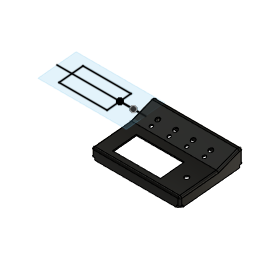
F24-Top (Autodesk Fusion 360 design; units mm, degrees)
Autodesk Fusion 360 part; units mm, degrees
sketch "Sketch1" plane through (0, 0, 0) normal (1, 0, 0) x (0, 1, 0)
  line L0 (49.5653, 19.5568) -> (20.1722, 19.5568)
  line L1 (-50.4347, -6.4432) -> (49.5653, -6.4432)
  line L2 (49.5653, 3.5568) -> (-50.4347, -6.4432)
  line L3 (20.1722, 19.5568) -> (20.1722, 28.5568)
  line L4 (44.5653, 26.5568) -> (43.5653, 26.5568)
  line L5 (-50.4347, 19.5568) -> (-50.4347, -6.4432)
  line L6 (20.1722, 19.5568) -> (10.0727, 15.6075)
  line L7 (49.5653, -6.4432) -> (-15.6066, -6.4432)
  line L8 (67.3511, 38.0053) -> (20.1722, 19.5568)
  line L9 (10.5451, 13.6448) -> (-45.4347, 8.0468)
  line L10 (43.5653, 26.5568) -> (10.5451, 13.6448)
  line L11 (20.1722, 28.5568) -> (49.5653, 28.5568)
  line L12 (44.5653, 3.0568) -> (44.5653, 26.5568)
  line L13 (-15.6066, -6.4432) -> (-15.6066, -63.0186)
  line L14 (49.5653, 19.5568) -> (-50.4347, 9.5568)
  line L15 (-45.4347, 8.0468) -> (-45.4347, -5.9432)
  line L16 (49.5653, 28.5568) -> (49.5653, 19.5568)
  line L17 (49.5653, 19.5568) -> (-50.4347, 19.5568)
  line L18 (49.5653, -6.4432) -> (49.5653, 19.5568)
  line L19 (49.5653, -63.0186) -> (49.5653, -6.4432)
  line L20 (-15.6066, -63.0186) -> (49.5653, -63.0186)
  line L21 (-15.6066, -6.4432) -> (-63.7664, -6.4432)
  line L22 (-63.7664, -6.4432) -> (-63.7664, -63.0262)
  line L23 (-63.7664, -63.0262) -> (-15.6066, -63.0262)
  line L24 (-15.6066, -63.0262) -> (-15.6066, -6.4432)
  line L25 (53.9927, 48.0645) -> (16.8652, 48.0645)
  line L26 (16.8652, 48.0645) -> (16.8652, 28.5568)
  line L27 (16.8652, 28.5568) -> (53.9927, 28.5568)
  line L28 (53.9927, 28.5568) -> (53.9927, 48.0645)
  point P0 (34.5128, -10.5651)
  dimension "d1" = 10
  dimension "d2" = 10
  dimension "d3" = 16
  dimension "d5" = 9
  dimension "d9" = 5
  dimension "d10" = 2
  dimension "d12" = 2
  dimension "d13" = 2
  dimension "d15" = 5
  dimension "d99" = 100
  dimension "d100" = 1
  dimension "d84" = 65.172
  constraint horizontal L17
  constraint vertical L5
  constraint horizontal L1
  constraint vertical L18
  constraint coincident L2.start L18
  constraint coincident L14.end L5
  constraint horizontal L0
  constraint vertical L3
  constraint horizontal L11
  constraint vertical L16
  constraint coincident L6.end L14
  constraint parallel L6 L8
  constraint coincident L12.start L2
  constraint vertical L12
  constraint perpendicular L4 L12
  constraint parallel L9 L14
  constraint coincident L15.end L2
  constraint perpendicular L1 L15
  constraint parallel L8 L10
  constraint horizontal L7
  constraint vertical L13
  constraint horizontal L20
  constraint vertical L19
  constraint horizontal L21
  constraint vertical L22
  constraint horizontal L23
  constraint vertical L24
  constraint horizontal L25
  constraint vertical L26
  constraint horizontal L27
  constraint vertical L28
  constraint coincident L3.end L27
  measures "d1" distance of L2.start L1.end
  measures "d2" distance of L5.start L14.end
  measures "d3" distance of L1.start L14.end
  measures "d5" distance of L0 L11
  measures "d9" distance of L12 L16
  measures "d10" distance of L4 L11
  measures "d12" distance of L8 L10
  measures "d13" distance of L9 L14
  measures "d15" distance of L5 L15
  measures "d99" distance of L5 L18
  measures "d100" distance of L4.end L12
  measures "d84" distance of L13 L19
extrude "Extrude1" add sketch "Sketch1" along normal blind 140 contours L0 L12 L14 L17 | L2 L12 L14 L18 | L0 L4 L8 L10 L11 L12 L16 L17 L27 | L0 L10 L12 L14 L17 | L0 L4 L10 L12 L17 | L2 L9 L10 L12 L14 L15 | L0 L6 L10 L14 L17 | L2 L5 L9 L10 L14 L15 picked at (46.232, 19.3901) picked at (46.232, 8.5568) picked at (47.8987, 24.8901) picked at (29.2269, 18.3197) picked at (37.9316, 21.8901) picked at (3.2253, 3.5861) picked at (15.8988, 17.1699) picked at (-48.768, 3.7201)
extrude "Extrude2" cut sketch "Sketch1" along normal blind 130 from surface at 5 contours L0 L10 L12 L14 L17 | L0 L4 L10 L12 L17 | L2 L9 L10 L12 L14 L15 picked at (29.2269, 18.3197) picked at (37.9316, 21.8901) picked at (3.2253, 3.5861)
sketch "Sketch2" plane through (0, -1.4456, 14.4557) normal (0, -0.099504, 0.995037) x (1, 0, 0)
  line L0 (0, 11.5757) -> (0, -49.2334)
  line L1 (0, -49.2334) -> (140, -49.2334)
  line L2 (140, -49.2334) -> (140, 11.5757)
  line L3 (140, 11.5757) -> (0, 11.5757)
  line L4 (23.5, -1.2334) -> (99.5, -1.2334)
  line L5 (99.5, -1.2334) -> (99.5, -39.2334)
  line L6 (99.5, -39.2334) -> (23.5, -39.2334)
  line L7 (23.5, -39.2334) -> (23.5, -1.2334)
  line L8 (0, -18.8289) -> (140, -18.8289)
  circle A0 centre (120.75, -18.8289) radius 3.5
  line L9 (99.5, -18.8289) -> (140, -18.8289)
  point P0 (99.5, -18.8289)
  dimension "d23" = 10
  dimension "d24" = 23.5
  dimension "d25" = 38
  dimension "d26" = 76
  dimension "d150" = 7
  constraint horizontal L4
  constraint vertical L5
  constraint horizontal L6
  constraint vertical L7
  constraint midpoint L0 L8.start
  constraint midpoint L2 L8.end
  constraint coincident L8 P0
  constraint coincident L5 P0
  constraint coincident L8 A0.centre
  constraint coincident P0 L9.start
  measures "d23" distance of L1 L6
  measures "d24" distance of L0 L7
  measures "d25" distance of L4 L6
  measures "d26" distance of L5 L7
  measures "d150" diameter of A0
extrude "Extrude3" cut sketch "Sketch2" against normal blind 5 contours L5 L6 L7 L8 | L4 L5 L7 L8 picked at (74.1667, -25.6304) picked at (48.8333, -7.0986)
sketch "Sketch3" plane through (0, 0, 0) normal (0, 0, 1) x (1, 0, 0)
  line L0 (130, -45.4347) -> (130, -40.4347)
  line L1 (135, 39.5653) -> (135, 44.5653)
  circle A0 centre (130, -40.4347) radius 5
  line L2 (130.0105, -37.1347) -> (127.1474, -38.7756)
  line L3 (132.8526, -42.0937) -> (132.8631, -38.7937)
  line L4 (135, -40.4347) -> (135, -45.4347)
  line L5 (135, -45.4347) -> (130, -45.4347)
  line L6 (130, 44.5653) -> (130, 39.5653)
  line L7 (135, 44.5653) -> (130, 44.5653)
  line L8 (130, 36.2653) -> (132.8579, 37.9153)
  circle A1 centre (130, -40.4347) radius 5
  line L9 (127.1369, -42.0756) -> (129.9895, -43.7346)
  line L10 (127.1421, 37.9153) -> (130, 36.2653)
  circle A2 centre (130, 39.5653) radius 2.5
  circle A3 centre (130, -40.4347) radius 3.3
  line L11 (132.8631, -38.7937) -> (130.0105, -37.1347)
  line L12 (127.1474, -38.7756) -> (127.1369, -42.0756)
  line L13 (132.8579, 37.9153) -> (132.8579, 41.2153)
  line L14 (130, 39.5653) -> (135, 39.5653)
  line L15 (132.8579, 41.2153) -> (130, 42.8653)
  line L16 (130, -40.4347) -> (135, -40.4347)
  line L17 (130, 42.8653) -> (127.1421, 41.2153)
  line L18 (127.1421, 41.2153) -> (127.1421, 37.9153)
  circle A4 centre (130, 39.5653) radius 3.3
  line L19 (10.0077, -37.1347) -> (7.146, -38.778)
  line L20 (7.146, -38.778) -> (7.1383, -42.078)
  line L21 (12.8617, -38.7914) -> (10.0077, -37.1347)
  line L22 (12.8579, 41.2153) -> (10, 42.8653)
  circle A5 centre (10, 39.5653) radius 3.3
  line L23 (7.1421, 41.2153) -> (7.1421, 37.9153)
  line L24 (12.854, -42.0914) -> (12.8617, -38.7914)
  line L25 (10, 44.5653) -> (10, 39.5653)
  circle A6 centre (10, -40.4347) radius 2.5
  circle A7 centre (10, -40.4347) radius 5
  line L26 (10, 42.8653) -> (7.1421, 41.2153)
  circle A8 centre (10, 39.5653) radius 2.5
  line L27 (5, 44.5653) -> (10, 44.5653)
  line L28 (7.1421, 37.9153) -> (10, 36.2653)
  line L29 (5, -45.4347) -> (10, -45.4347)
  circle A9 centre (130, 39.5653) radius 5
  line L30 (10, -45.4347) -> (10, -40.4347)
  line L31 (7.1383, -42.078) -> (9.9923, -43.7347)
  line L32 (10, 36.2653) -> (12.8579, 37.9153)
  line L33 (5, 39.5653) -> (5, 44.5653)
  line L34 (9.9923, -43.7347) -> (12.854, -42.0914)
  line L35 (10, -40.4347) -> (5, -40.4347)
  circle A10 centre (130, -40.4347) radius 2.5
  line L36 (129.9895, -43.7346) -> (132.8526, -42.0937)
  circle A11 centre (10, 39.5653) radius 5
  circle A12 centre (10, -40.4347) radius 3.3
  line L37 (5, -40.4347) -> (5, -45.4347)
  line L38 (10, 39.5653) -> (5, 39.5653)
  line L39 (12.8579, 37.9153) -> (12.8579, 41.2153)
  line L40 (5, -45.4347) -> (135, -45.4347)
  line L41 (135, -45.4347) -> (135, 44.5653)
  line L42 (5, 44.5653) -> (5, -45.4347)
  line L43 (135, 44.5653) -> (5, 44.5653)
  point P0 (10, -40.4347)
  point P1 (130, 39.5653)
  point P2 (130, -40.4347)
  point P3 (10, 39.5653)
  point P4 (135, 44.5653)
  point P5 (5, 44.5653)
  point P6 (5, 44.5653)
  point P7 (5, -45.4347)
  point P8 (135, 44.5653)
  point P9 (135, -45.4347)
  point P10 (135, -45.4347)
  point P11 (5, -45.4347)
  dimension "d60" = 5
  dimension "d61" = 5
  dimension "d62" = 5
  dimension "d63" = 5
  dimension "d64" = 5
  dimension "d65" = 5
  dimension "d66" = 5
  dimension "d67" = 5
  dimension "d68" = 10
  dimension "d69" = 10
  dimension "d70" = 10
  dimension "d71" = 10
  dimension "d72" = 6.6
  dimension "d73" = 6.6
  dimension "d74" = 6.6
  dimension "d75" = 6.6
  dimension "d89" = 5
  dimension "d90" = 5
  dimension "d91" = 5
  dimension "d92" = 5
  constraint coincident P11 P7
  constraint horizontal L29
  constraint vertical L30
  constraint horizontal L35
  constraint vertical L37
  constraint coincident P6 P5
  constraint coincident P8 P4
  constraint coincident P10 P9
  constraint horizontal L27
  constraint vertical L25
  constraint horizontal L38
  constraint vertical L33
  constraint horizontal L7
  constraint vertical L6
  constraint horizontal L14
  constraint vertical L1
  constraint horizontal L5
  constraint vertical L0
  constraint horizontal L16
  constraint vertical L4
  constraint coincident P3 A5.centre
  constraint coincident P1 L6.end
  constraint coincident P2 L0.end
  constraint coincident P0 A6.centre
  constraint concentric A5 A11
  constraint concentric A4 A9
  constraint concentric A0 A1
  constraint concentric A1 A3
  constraint concentric A7 A12
  constraint coincident L22.end L25
  constraint coincident L22.end A5
  constraint coincident L15.end L6
  constraint coincident L15.end A4
  constraint coincident L2.start A3
  constraint coincident L19.start A12
  constraint concentric A8 A11
  constraint concentric A1 A10
  constraint concentric A6 A7
  constraint tangent A0 L40
  constraint tangent A0 L41
  constraint tangent A7 L40
  constraint tangent A7 L42
  constraint tangent A11 L43
  constraint tangent A9 L43
  constraint tangent A9 L41
  constraint tangent A11 L42
  measures "d60" distance of L29 L35
  measures "d61" distance of L30 L37
  measures "d62" distance of L27 L38
  measures "d63" distance of L25 L33
  measures "d64" distance of L1 L6
  measures "d65" distance of L7 L14
  measures "d66" distance of L5 L16
  measures "d67" distance of L0 L4
  measures "d68" diameter of A11
  measures "d69" diameter of A9
  measures "d70" diameter of A0
  measures "d71" diameter of A7
  measures "d72" diameter of A12
  measures "d73" diameter of A5
  measures "d74" diameter of A4
  measures "d75" diameter of A3
  measures "d89" diameter of A8
  measures "d90" diameter of A2
  measures "d91" diameter of A10
  measures "d92" diameter of A6
extrude "Extrude4" add sketch "Sketch3" along normal blind 10 and the other way blind 6 contours L0 A0 A1 A3 L16 | L0 A0 A1 A3 L16 | A0 L4 L5 A1 L40 L41 | L0 A3 L36 | A7 L29 L37 L40 L42 | A7 L30 L35 A12 | A7 L30 L35 A12 | L0 L2 L3 L9 L11 L12 L16 A10 L36 | L0 L3 L16 A10 L36 | L9 A3 | L3 A3 L16 | L3 A3 L16 | L20 A6 L30 L31 L34 L35 | L19 L20 L21 L24 A6 L30 L34 L35 | L34 A12 | L0 L16 A10 | L0 L16 A10 | A3 L12 | A3 L11 | L20 L35 A12 | L20 L35 A12 | A6 L30 L35 | A6 L30 L35 | L31 A12 | L24 A12 | L2 A3 | L19 A12 | L21 A12 picked at (133.8468, -38.2491) picked at (133.869, -42.5811) picked at (134.0177, -44.4523) picked at (131.809, -42.7738) picked at (5.9823, -44.4523) picked at (6.5428, -37.6743) picked at (6.1279, -42.5759) picked at (132.7044, -39.6458) picked at (132.7031, -41.2225) picked at (128.18, -42.7647) picked at (133.1431, -40.5791) picked at (133.1433, -40.2919) picked at (7.2939, -41.2172) picked at (7.2997, -39.6368) picked at (11.81, -42.7745) picked at (128.9774, -41.745) picked at (130.3534, -42.0591) picked at (127.0695, -40.8273) picked at (131.1932, -37.6015) picked at (6.8569, -40.2904) picked at (6.8567, -40.5776) picked at (8.4529, -39.8275) picked at (8.3418, -40.5533) picked at (8.877, -43.1697) picked at (12.9223, -40.02) picked at (128.4145, -37.8008) picked at (8.4337, -37.8721) picked at (11.6499, -37.7561)
extrude "Extrude5" add sketch "Sketch3" along normal blind 32 from surface at 2 contours L1 L7 A9 L41 L43 | L6 L14 A4 A9 | L6 L14 A4 A9 | L13 L14 A4 | L13 L14 A4 | L27 L33 A11 L42 L43 | A5 L25 A11 L38 | A5 L25 A11 L38 | L6 A2 L13 L14 L15 | L6 L8 L10 A2 L13 L14 L17 L18 | L15 A4 | L8 A4 | L17 A4 | A5 L23 L38 | A5 L23 L38 | L6 A2 L14 | L6 A2 L14 | L10 A4 | L18 A4 | L22 A5 | A5 L26 | L22 L23 L25 A8 L28 L32 L38 L39 | L23 L25 L26 A8 L38 | A5 L28 | A5 L39 | L25 A8 L38 | L25 A8 L38 | A5 L32 picked at (134.0177, 43.583) picked at (133.8451, 37.3768) picked at (133.8708, 41.7088) picked at (133.1432, 39.4218) picked at (133.1432, 39.7089) picked at (5.9823, 43.583) picked at (7.5079, 35.91) picked at (6.1292, 41.7088) picked at (132.7048, 40.3501) picked at (132.7027, 38.7734) picked at (131.1842, 42.4023) picked at (131.1166, 36.8276) picked at (128.7231, 42.2665) picked at (6.8568, 39.4218) picked at (6.8568, 39.7089) picked at (130.3534, 41.1898) picked at (130.5214, 37.9871) picked at (128.8834, 36.8276) picked at (127.0708, 39.1635) picked at (11.2255, 42.4628) picked at (8.7745, 42.4628) picked at (7.2984, 38.7697) picked at (7.2952, 40.3501) picked at (8.1874, 37.2295) picked at (12.9215, 39.1444) picked at (8.3426, 39.4411) picked at (8.5409, 40.3621) picked at (11.8126, 37.2295)
extrude "Extrude6" cut sketch "Sketch3" along normal blind 8 and the other way blind 12 contours L0 L16 A10 | L0 L16 A10 | A6 L30 L35 | A6 L30 L35 picked at (128.9774, -41.745) picked at (130.3534, -42.0591) picked at (8.4529, -39.8275) picked at (8.3418, -40.5533)
extrude "Extrude7" cut sketch "Sketch3" along normal blind 22 contours L6 A2 L14 | L6 A2 L14 | L25 A8 L38 | L25 A8 L38 picked at (130.3534, 41.1898) picked at (130.5214, 37.9871) picked at (8.3426, 39.4411) picked at (8.5409, 40.3621)
extrude "Extrude8" cut sketch "Sketch3" against normal blind 6 from surface at -2.25 contours L0 L2 L3 L9 L11 L12 L16 A10 L36 | L0 L3 L16 A10 L36 | L20 A6 L30 L31 L34 L35 | L19 L20 L21 L24 A6 L30 L34 L35 | L0 L16 A10 | L0 L16 A10 | A6 L30 L35 | A6 L30 L35 picked at (132.7044, -39.6458) picked at (132.7031, -41.2225) picked at (7.2939, -41.2172) picked at (7.2997, -39.6368) picked at (128.9774, -41.745) picked at (130.3534, -42.0591) picked at (8.4529, -39.8275) picked at (8.3418, -40.5533)
extrude "Extrude9" cut sketch "Sketch3" along normal blind 3.75 from surface at 2 contours L6 A2 L13 L14 L15 | L6 L8 L10 A2 L13 L14 L17 L18 | L6 A2 L14 | L6 A2 L14 | L22 L23 L25 A8 L28 L32 L38 L39 | L23 L25 L26 A8 L38 | L25 A8 L38 | L25 A8 L38 picked at (132.7048, 40.3501) picked at (132.7027, 38.7734) picked at (130.3534, 41.1898) picked at (130.5214, 37.9871) picked at (7.2984, 38.7697) picked at (7.2952, 40.3501) picked at (8.3426, 39.4411) picked at (8.5409, 40.3621)
chamfer "Chamfer1" distance 5 distance2 2.5 1 edges at (127.6692, -41.3387, 8) measured on face at (130.6771, -42.8412, 1.1667)
chamfer "Chamfer2" distance 5 distance2 2.5 1 edges at (127.6692, 38.6613, 22) measured on face at (129.8993, 37.0674, 11.1667)
chamfer "Chamfer3" distance 5 distance2 2.5 1 edges at (7.6692, 38.6613, 22) measured on face at (12.4919, 39.7665, 16.5833)
chamfer "Chamfer4" distance 5 distance2 2.5 1 edges at (7.6692, -41.3387, 8) measured on face at (12.4969, -40.31, 1.1667)
extrude "Extrude10" cut sketch "Sketch1" along normal blind 140 contours L1 L2 L7 L18 L21 | L1 L7 L13 L19 L20 L24 | L1 L13 L21 L22 L23 L24 picked at (26.1747, -3.2766) picked at (27.8414, -44.1602) picked at (-43.2692, -44.1627)
extrude "Extrude11" cut sketch "Sketch1" along normal blind 140 contours L8 L11 L27 L28 | L8 L11 L25 L26 L27 L28 | L3 L8 L11 L27 picked at (52.5169, 29.9651) picked at (38.0154, 41.562) picked at (27.8442, 25.5568)
sketch "Sketch4" plane through (0, 49.5653, 0) normal (0, 1, 0) x (-1, 0, 0)
  line L0 (0, 3.5568) -> (0, 28.5568)
  line L1 (0, 28.5568) -> (-140, 28.5568)
  line L2 (-140, 28.5568) -> (-140, 3.5568)
  line L3 (-140, 3.5568) -> (0, 3.5568)
  line L4 (-39.5, 13.5568) -> (-28, 13.5568)
  line L5 (-28, 13.5568) -> (-28, 5.5568)
  line L6 (-28, 5.5568) -> (-39.5, 5.5568)
  line L7 (-39.5, 5.5568) -> (-39.5, 13.5568)
  dimension "d103" = 8
  dimension "d104" = 11.5
  dimension "d105" = 28
  dimension "d106" = 10
  constraint horizontal L4
  constraint vertical L5
  constraint horizontal L6
  constraint vertical L7
  measures "d103" distance of L4 L6
  measures "d104" distance of L5 L7
  measures "d105" distance of L0 L5
  measures "d106" distance of L3 L4
extrude "Extrude12" cut sketch "Sketch4" against normal blind 10 contours L4 L5 L6 L7 picked at (-35.6667, 8.2234)
fillet "Fillet1" radius 2.5 4 edges at (28, 47.0653, 5.5568) (39.5, 47.0653, 5.5568) (28, 47.0653, 13.5568) (39.5, 47.0653, 13.5568)
ref_plane "WorkPlane1" through (0, 0, 15.6) normal (0, 0, 1) x (1, 0, 0)
sketch "Sketch6" plane through (0, 0, 15.6) normal (0, 0, 1) x (1, 0, 0)
  line L0 (0, -50.4347) -> (140, -50.4347)
  line L1 (140, -50.4347) -> (140, 49.5653)
  line L2 (140, 49.5653) -> (0, 49.5653)
  line L3 (0, 49.5653) -> (0, -50.4347)
  line L4 (5.25, -50.4347) -> (0, -45.1847)
  line L5 (134.75, -50.4347) -> (140, -45.1847)
  line L6 (140, 44.3153) -> (134.75, 49.5653)
  line L7 (5.25, 49.5653) -> (0, 44.3153)
  line L8 (140, -50.4347) -> (134.75, -50.4347)
  line L9 (134.75, -50.4347) -> (140, -50.4347)
  line L10 (140, -50.4347) -> (140, -45.2582)
  point P0 (0, -50.4347)
  point P1 (0, 49.5653)
  point P2 (140, 49.5653)
  point P3 (140, -50.4347)
  dimension "d120" = 5.25
  dimension "d121" = 5.25
  dimension "d122" = 5.25
  dimension "d123" = 5.25
  dimension "d124" = 5.25
  dimension "d125" = 5.25
  dimension "d126" = 5.25
  dimension "d127" = 5.25
  constraint horizontal L0
  constraint vertical L1
  constraint horizontal L2
  constraint vertical L3
  constraint coincident L0 P0
  constraint coincident L3 P1
  constraint coincident L2 P2
  constraint coincident L1 P3
  constraint coincident L0 L4.start
  constraint coincident L3 L4.end
  constraint coincident L0 L5.start
  constraint coincident L1 L5.end
  constraint coincident L1 L6.start
  constraint coincident L2 L6.end
  constraint perpendicular L5 L6
  constraint coincident L2 L7.start
  constraint coincident L3 L7.end
  constraint perpendicular L6 L7
  constraint coincident P3 L0.end
  constraint coincident L1 L10.end
  constraint perpendicular L9 L10
  measures "d120" horizontal distance of L7.start L7.end
  measures "d121" distance of P1 L7.end
  measures "d122" distance of P0 L4.end
  measures "d123" distance of P0 L4.start
  measures "d124" distance of P3 L5.start
  measures "d125" distance of P3 L5.end
  measures "d126" distance of P2 L6.start
  measures "d127" distance of P2 L6.end
extrude "Extrude13" cut sketch "Sketch6" against normal blind 9 from surface at -18.547 contours L0 L3 L4 | L0 L1 L5 L8 L9 L10 picked at (1.75, -48.6847) picked at (138.25, -48.7092)
extrude "Extrude14" cut sketch "Sketch6" against normal blind 10 from surface at -8.457 contours L2 L3 L7 | L1 L2 L6 picked at (1.75, 47.8153) picked at (138.25, 47.8153)
fillet "Fillet2" radius 3 4 edges at (0, 49.5653, 17.8499) (0, -50.4347, 3.3049) (140, -50.4347, 3.3049) (140, 49.5653, 17.8499)
sketch "Sketch7" plane through (0, -3.9577, 10.1212) normal (0, -0.36418, 0.931329) x (1, 0, 0)
  line L0 (0, 50.6222) -> (0, 15.0649)
  line L1 (0, 15.0649) -> (140, 15.0649)
  line L2 (140, 15.0649) -> (140, 50.6222)
  line L3 (140, 50.6222) -> (0, 50.6222)
  circle A0 centre (28, 32.8436) radius 3.5
  circle A1 centre (56, 32.8436) radius 3.5
  circle A2 centre (84, 32.8436) radius 3.5
  circle A3 centre (112, 32.8436) radius 3.5
  line L4 (0, 32.8436) -> (140, 32.8436)
  line L5 (0, 32.8436) -> (0, 15.0649)
  line L6 (140, 32.8436) -> (140, 15.0649)
  line L7 (0, 21.9542) -> (140, 21.9542)
  circle A4 centre (28, 21.9542) radius 2.65
  circle A5 centre (56, 21.9542) radius 2.65
  circle A6 centre (84, 21.9542) radius 2.65
  circle A7 centre (112, 21.9542) radius 2.65
  line L8 (0, 50.6222) -> (0, 32.8436)
  line L9 (140, 50.6222) -> (140, 32.8436)
  point P0 (0, 32.8436)
  point P1 (140, 32.8436)
  point P2 (0, 15.0649)
  point P3 (140, 15.0649)
  dimension "d136" = 28
  dimension "d137" = 28
  dimension "d138" = 28
  dimension "d139" = 28
  dimension "d140" = 7
  dimension "d141" = 7
  dimension "d142" = 7
  dimension "d143" = 7
  dimension "d144" = 5.3
  dimension "d145" = 5.3
  dimension "d146" = 5.3
  dimension "d147" = 5.3
  constraint midpoint L0 P0
  constraint midpoint L2 P1
  constraint coincident P0 L4.start
  constraint coincident P1 L4.end
  constraint coincident A0.centre L4
  constraint coincident A1.centre L4
  constraint coincident A2.centre L4
  constraint coincident A3.centre L4
  constraint coincident L0.end L1.start
  constraint coincident L1.end L2.start
  constraint coincident P2 L0.end
  constraint coincident P3 L1.end
  constraint coincident L7 A4.centre
  constraint coincident L7 A5.centre
  constraint coincident L7 A6.centre
  constraint coincident L7 A7.centre
  constraint coincident L0.start L3.end
  constraint coincident L2.end L3.start
  measures "d136" distance of A0.centre P0
  measures "d137" distance of A0.centre A1.centre
  measures "d138" distance of A1.centre A2.centre
  measures "d139" distance of A2.centre A3.centre
  measures "d140" diameter of A0
  measures "d141" diameter of A1
  measures "d142" diameter of A2
  measures "d143" diameter of A3
  measures "d144" diameter of A4
  measures "d145" diameter of A5
  measures "d146" diameter of A6
  measures "d147" diameter of A7
extrude "Extrude15" cut sketch "Sketch7" against normal blind 3 contours A0 L4 | A0 L4 | L7 A4 | L7 A4 | A3 L4 | A3 L4 | A1 L4 | A1 L4 | L7 A7 | L7 A7 | L7 A5 | L7 A5 | A2 L4 | A2 L4 | L7 A6 | L7 A6 picked at (28.0872, 31.6802) picked at (28.0872, 34.007) picked at (28.7298, 22.7151) picked at (28.6382, 20.8804) picked at (111.4167, 35.1683) picked at (112.8552, 31.3623) picked at (56.0872, 31.6802) picked at (56.0872, 34.007) picked at (111.1943, 21.4393) picked at (112.7959, 22.3375) picked at (55.3324, 23.4517) picked at (55.5191, 20.9289) picked at (83.2658, 34.855) picked at (84.8552, 31.3623) picked at (84.066, 20.8101) picked at (84.6284, 23.1598)
extrude "Extrude16" cut sketch "Sketch2" against normal blind 3 contours L8 A0 L9 | L8 A0 L9 picked at (121.6052, -20.3102) picked at (120.3238, -16.4284)
fillet "Fillet3" radius 3 12 edges at (0, -18.681, 12.7321) (0.8787, -49.556, 9.6446) (70, -50.4347, 9.5568) (139.1213, -49.556, 9.6446) (140, -18.681, 12.7321) (140, 26.6304, 22.0821) (0, 44.8768, 28.5568) (0.8787, 48.6867, 28.5568) (70, 49.5653, 28.5568) (139.1213, 48.6867, 28.5568) (140, 44.8768, 28.5568) (0, 26.6304, 22.0821)
move_body "Déplacer1" bodies 1 to x (1, 0, 0) y (0, 1, 0) z (0, 0, 1) at (130, -45.4347, -5.9432)
equation "d128 = -21.547 mm + 3 mm"
equation "d133 = -11.457 mm + 3 mm"
equation "d136 = ( 140 / 5 ) * 1 mm"
